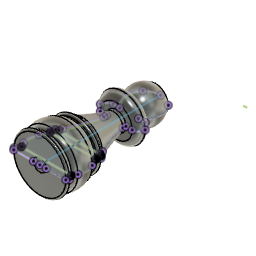
Pawn v1 (Autodesk Fusion 360 design; units mm, degrees)
Autodesk Fusion 360 part; units mm, degrees
sketch "SVG" plane through (0, 0, 0) normal (0, 0, 1) x (1, 0, 0)
  line L0 (6.638277, 6.628661) -> (13.5992, 6.628661)
  spline S0 degree 3 poles (13.5992, 6.628661) (13.764035, 6.697718) (13.883627, 6.821014) (13.840499, 7.032678) knots 0 0 0 0 1 1 1 1
  spline S1 degree 3 poles (13.840499, 7.032678) (13.797107, 7.245932) (13.689951, 7.340653) (13.552897, 7.384045) knots 0 0 0 0 1 1 1 1
  line L1 (13.552897, 7.384045) -> (6.732998, 7.384045)
  spline S2 degree 3 poles (6.732998, 7.384045) (6.567368, 7.312607) (6.482173, 7.158356) (6.47741, 6.931344) knots 0 0 0 0 1 1 1 1
  spline S3 degree 3 poles (6.47741, 6.931344) (6.473706, 6.755926) (6.539058, 6.6702) (6.638277, 6.628661) knots 0 0 0 0 1 1 1 1
  line L2 (6.393008, 2.442159) -> (13.837325, 2.442159)
  spline S4 degree 3 poles (13.837325, 2.442159) (14.039467, 2.558577) (14.139479, 2.79538) (14.237375, 3.040645) knots 0 0 0 0 1 1 1 1
  spline S5 degree 3 poles (14.237375, 3.040645) (14.557785, 3.840217) (14.452481, 4.624972) (14.138157, 5.390409) knots 0 0 0 0 1 1 1 1
  spline S6 degree 3 poles (14.138157, 5.390409) (13.977819, 5.780933) (13.813512, 6.179661) (13.492838, 6.478375) knots 0 0 0 0 1 1 1 1
  line L3 (13.492838, 6.478375) -> (6.728764, 6.478375)
  spline S7 degree 3 poles (6.728764, 6.478375) (6.705217, 6.464883) (6.683256, 6.447156) (6.663677, 6.421224) knots 0 0 0 0 1 1 1 1
  spline S8 degree 3 poles (6.663677, 6.421224) (5.92496, 5.438032) (5.450033, 4.392133) (5.901942, 3.132984) knots 0 0 0 0 1 1 1 1
  spline S9 degree 3 poles (5.901942, 3.132984) (6.059633, 2.693513) (6.152237, 2.513332) (6.393008, 2.442159) knots 0 0 0 0 1 1 1 1
  line L4 (13.857169, 2.29214) -> (6.251721, 2.29214)
  spline S10 degree 3 poles (6.251721, 2.29214) (5.976554, 2.202712) (5.81754, 1.928072) (5.850083, 1.583588) knots 0 0 0 0 1 1 1 1
  spline S11 degree 3 poles (5.850083, 1.583588) (5.886596, 1.196237) (6.201185, 1.374302) (6.371577, 1.372187) knots 0 0 0 0 1 1 1 1
  spline S12 degree 3 poles (6.371577, 1.372187) (7.901398, 1.354459) (9.431483, 1.363721) (10.961304, 1.365307) knots 0 0 0 0 1 1 1 1
  spline S13 degree 3 poles (10.961304, 1.365307) (11.987094, 1.365836) (13.013413, 1.37404) (14.039202, 1.365307) knots 0 0 0 0 1 1 1 1
  spline S14 degree 3 poles (14.039202, 1.365307) (14.29479, 1.362663) (14.34903, 1.449976) (14.296906, 1.687833) knots 0 0 0 0 1 1 1 1
  spline S15 degree 3 poles (14.296906, 1.687833) (14.222559, 2.028881) (14.119106, 2.199272) (13.857169, 2.29214) knots 0 0 0 0 1 1 1 1
  spline S16 degree 3 poles (11.453165, 12.878913) (11.390459, 13.146936) (11.38014, 13.267322) (11.475919, 13.320767) knots 0 0 0 0 1 1 1 1
  line L5 (11.475919, 13.320767) -> (12.455935, 13.320767)
  spline S17 degree 3 poles (12.455935, 13.320767) (13.013677, 13.320767) (13.46585, 13.77294) (13.46585, 14.330944) knots 0 0 0 0 1 1 1 1
  spline S18 degree 3 poles (13.46585, 14.330944) (13.46585, 14.888686) (13.013677, 15.341122) (12.455935, 15.341122) knots 0 0 0 0 1 1 1 1
  line L6 (12.455935, 15.341122) -> (11.438877, 15.341122)
  spline S19 degree 3 poles (11.438877, 15.341122) (11.429352, 15.344295) (11.420092, 15.346943) (11.410831, 15.350383) knots 0 0 0 0 1 1 1 1
  spline S20 degree 3 poles (11.410831, 15.350383) (13.075854, 16.539684) (12.898053, 18.449185) (11.933647, 19.477354) knots 0 0 0 0 1 1 1 1
  spline S21 degree 3 poles (11.933647, 19.477354) (11.002579, 20.469806) (9.249979, 20.579873) (8.185031, 19.460684) knots 0 0 0 0 1 1 1 1
  spline S22 degree 3 poles (8.185031, 19.460684) (7.351328, 18.58465) (6.960539, 16.736268) (8.722399, 15.341122) knots 0 0 0 0 1 1 1 1
  line L7 (8.722399, 15.341122) -> (7.647133, 15.341122)
  spline S23 degree 3 poles (7.647133, 15.341122) (7.089391, 15.341122) (6.636953, 14.888682) (6.636953, 14.330944) knots 0 0 0 0 1 1 1 1
  spline S24 degree 3 poles (6.636953, 14.330944) (6.636953, 13.77294) (7.089391, 13.320767) (7.647133, 13.320767) knots 0 0 0 0 1 1 1 1
  line L8 (7.647133, 13.320767) -> (8.59831, 13.320767)
  spline S25 degree 3 poles (8.59831, 13.320767) (8.788545, 13.257794) (8.759176, 13.091901) (8.647258, 12.651105) knots 0 0 0 0 1 1 1 1
  spline S26 degree 3 poles (8.647258, 12.651105) (8.233978, 11.020479) (7.806147, 9.394085) (7.164532, 7.83516) knots 0 0 0 0 1 1 1 1
  spline S27 degree 3 poles (7.164532, 7.83516) (7.101826, 7.683288) (7.115584, 7.616613) (7.183318, 7.58063) knots 0 0 0 0 1 1 1 1
  line L9 (7.183318, 7.58063) -> (13.14782, 7.58063)
  spline S28 degree 3 poles (13.14782, 7.58063) (13.248626, 7.655242) (13.202325, 7.751287) (13.083791, 8.027247) knots 0 0 0 0 1 1 1 1
  spline S29 degree 3 poles (13.083791, 8.027247) (12.407252, 9.599931) (11.845277, 11.211242) (11.453165, 12.878913) knots 0 0 0 0 1 1 1 1
  spline S30 degree 3 poles (18.34265, 25.31671) (18.224382, 25.33867) (18.094471, 25.302422) (17.970911, 25.289459) knots 0 0 0 0 1 1 1 1
  line L10 (9.96745, 20.259532) -> (9.96745, 1.363549)
  constraint perpendicular L4 L10
revolve "Revolve1" add sketch "SVG" angle 360 about axis through (9.96745, 20.259532, 0) along (0, -1, 0) contours L0 S0 S1 L1 L10 | L2 S4 S5 S6 L3 L10 | L4 S12 S13 S14 S15 L10 | S16 L5 S17 S18 L6 S19 S20 S21 L9 S28 S29 L10 picked at (12.373182, 6.880456) picked at (11.357685, 4.770315) picked at (11.595308, 1.983196) picked at (11.737686, 8.675112) makes body 1 at (11.280191, 6.628661, 0.862374) makes body 2 at (5.788284, 4.774023, -1.289102) makes body 3 at (12.419788, 9.613463, -0.369631) makes body 4 at (12.99814, 1.369306, -0.303266)
sketch "Pion" plane through (0, 0, 0) normal (0, 0, 1) x (1, 0, 0)
  spline S0 degree 3 poles (14.296906, 1.687833) (14.269631, 1.812951) (14.236651, 1.924427) (14.15614, 2.076533) (14.116832, 2.129723) (14.009728, 2.224115) (13.941741, 2.262156) (13.857169, 2.29214) knots -0.08939975 -0.08939975 -0.08939975 -0.08939975 -0.0516416 -0.0516416 -0.02691914 -0.02691914 0 0 0 0
  line L0 (13.857169, 2.29214) -> (6.077731, 2.29214)
  spline S1 degree 3 poles (6.077731, 2.29214) (6.018123, 2.271007) (5.960583, 2.243682) (5.861134, 2.172033) (5.821359, 2.131321) (5.719625, 1.986228) (5.675175, 1.858392) (5.637994, 1.687833) knots -0.10663916 -0.10663916 -0.10663916 -0.10663916 -0.07847511 -0.07847511 -0.05236952 -0.05236952 0 0 0 0
  spline S2 degree 3 poles (5.637994, 1.687833) (5.620994, 1.610259) (5.615328, 1.548816) (5.627557, 1.483197) (5.633268, 1.465739) (5.651293, 1.434659) (5.662703, 1.421924) (5.693629, 1.398463) (5.714663, 1.388482) (5.780478, 1.36961) (5.831783, 1.364646) (5.895698, 1.365307) knots -0.07987643 -0.07987643 -0.07987643 -0.07987643 -0.05202481 -0.05202481 -0.0414749 -0.0414749 -0.03139166 -0.03139166 -0.01917533 -0.01917533 0 0 0 0
  spline S3 degree 3 poles (5.895698, 1.365307) (6.408638, 1.369674) (6.921725, 1.369806) (7.947679, 1.367755) (8.460684, 1.365572) (8.973595, 1.365307) knots -0.30771325 -0.30771325 -0.30771325 -0.30771325 -0.15387332 -0.15387332 0 0 0 0
  spline S4 degree 3 poles (8.973595, 1.365307) (9.139235, 1.365136) (9.304876, 1.364874) (9.635567, 1.364259) (9.800634, 1.363907) (9.966264, 1.363551) (9.966857, 1.36355) (9.96745, 1.363549) knots -0.09919894 -0.09919894 -0.09919894 -0.09919894 -0.04951132 -0.04951132 0 0 0.00017787 0.00017787 0.00017787 0.00017787
  spline S5 degree 3 poles (9.96745, 1.363549) (9.968043, 1.36355) (9.968636, 1.363551) (10.134266, 1.363907) (10.299333, 1.364259) (10.630023, 1.364874) (10.795665, 1.365136) (10.961304, 1.365307) knots -0.09938539 -0.09938539 -0.09938539 -0.09938539 -0.09920751 -0.09920751 -0.04969191 -0.04969191 0 0 0 0
  spline S6 degree 3 poles (10.961304, 1.365307) (11.474215, 1.365572) (11.987221, 1.367755) (13.013175, 1.369806) (13.526262, 1.369674) (14.039202, 1.365307) knots -0.30780865 -0.30780865 -0.30780865 -0.30780865 -0.15388763 -0.15388763 0 0 0 0
  spline S7 degree 3 poles (14.039202, 1.365307) (14.074327, 1.364944) (14.112195, 1.366212) (14.176578, 1.37548) (14.203328, 1.382224) (14.242851, 1.40008) (14.258087, 1.409699) (14.283678, 1.4347) (14.293225, 1.449053) (14.308742, 1.485627) (14.313419, 1.50931) (14.316324, 1.578403) (14.309938, 1.628363) (14.296906, 1.687833) knots -0.08001679 -0.08001679 -0.08001679 -0.08001679 -0.06355834 -0.06355834 -0.04975587 -0.04975587 -0.03990536 -0.03990536 -0.03027504 -0.03027504 -0.01826445 -0.01826445 0 0 0 0
  spline S8 degree 3 poles (14.138157, 5.390409) (14.053933, 5.595547) (13.968609, 5.802964) (13.759865, 6.176143) (13.642707, 6.33877) (13.492838, 6.478375) knots -0.12796857 -0.12796857 -0.12796857 -0.12796857 -0.06144539 -0.06144539 0 0 0 0
  line L1 (13.492838, 6.478375) -> (6.442062, 6.478375)
  spline S9 degree 3 poles (6.442062, 6.478375) (6.284165, 6.331292) (6.162768, 6.15886) (5.95807, 5.782979) (5.876907, 5.58566) (5.796743, 5.390409) knots -0.12807049 -0.12807049 -0.12807049 -0.12807049 -0.06332025 -0.06332025 0 0 0 0
  spline S10 degree 3 poles (5.796743, 5.390409) (5.62307, 4.967483) (5.506569, 4.522493) (5.500445, 3.709827) (5.565678, 3.369664) (5.697524, 3.040645) knots -0.24362958 -0.24362958 -0.24362958 -0.24362958 -0.10633604 -0.10633604 0 0 0 0
  spline S11 degree 3 poles (5.697524, 3.040645) (5.766746, 2.86722) (5.837072, 2.697867) (5.988113, 2.520503) (6.038504, 2.476179) (6.097575, 2.442159) knots -0.06988605 -0.06988605 -0.06988605 -0.06988605 -0.02044994 -0.02044994 0 0 0 0
  line L2 (6.097575, 2.442159) -> (13.837325, 2.442159)
  spline S12 degree 3 poles (13.837325, 2.442159) (13.887664, 2.47115) (13.931836, 2.507702) (14.011586, 2.59368) (14.046091, 2.642386) (14.138963, 2.797517) (14.188442, 2.918051) (14.237375, 3.040645) knots -0.07769775 -0.07769775 -0.07769775 -0.07769775 -0.05882377 -0.05882377 -0.03959964 -0.03959964 0 0 0 0
  spline S13 degree 3 poles (14.237375, 3.040645) (14.314635, 3.233444) (14.369844, 3.432124) (14.43123, 3.833543) (14.438707, 4.030388) (14.399622, 4.629398) (14.290617, 5.019141) (14.138157, 5.390409) knots -0.24206707 -0.24206707 -0.24206707 -0.24206707 -0.17982962 -0.17982962 -0.12040588 -0.12040588 0 0 0 0
  line L3 (6.097575, 2.442159) -> (6.077731, 2.29214)
  line L4 (13.837325, 2.442159) -> (13.857169, 2.29214)
  spline S14 degree 3 poles (9.96745, 20.259532) (9.966566, 20.259564) (9.965682, 20.259595) (9.749904, 20.267162) (9.534261, 20.248772) (9.115206, 20.161638) (8.911934, 20.093397) (8.450603, 19.871433) (8.205829, 19.695418) (8.001252, 19.477354) knots -0.21837472 -0.21837472 -0.21837472 -0.21837472 -0.21810941 -0.21810941 -0.15361398 -0.15361398 -0.08970139 -0.08970139 0 0 0 0
  spline S15 degree 3 poles (8.001252, 19.477354) (7.832849, 19.297816) (7.690511, 19.093672) (7.462424, 18.650745) (7.377782, 18.410828) (7.261314, 17.841501) (7.254004, 17.509559) (7.366737, 16.849565) (7.488608, 16.533131) (7.888418, 15.889507) (8.18373, 15.593482) (8.524069, 15.350383) knots -0.47792048 -0.47792048 -0.47792048 -0.47792048 -0.40348961 -0.40348961 -0.32738532 -0.32738532 -0.22800437 -0.22800437 -0.12547317 -0.12547317 0 0 0 0
  spline S16 degree 3 poles (8.524069, 15.350383) (8.519455, 15.348669) (8.514853, 15.347156) (8.505499, 15.344169) (8.500762, 15.342701) (8.496023, 15.341122) knots -0.00301721 -0.00301721 -0.00301721 -0.00301721 -0.00149859 -0.00149859 0 0 0 0
  line L5 (8.496023, 15.341122) -> (7.478964, 15.341122)
  spline S17 degree 3 poles (7.478964, 15.341122) (7.408737, 15.341122) (7.338867, 15.333949) (7.203545, 15.305485) (7.138597, 15.284743) (6.954326, 15.204474) (6.84409, 15.127633) (6.662246, 14.938978) (6.590998, 14.829587) (6.49371, 14.589263) (6.46905, 14.461195) (6.46905, 14.330944) knots -0.15943999 -0.15943999 -0.15943999 -0.15943999 -0.13834264 -0.13834264 -0.1178842 -0.1178842 -0.07792732 -0.07792732 -0.03907516 -0.03907516 0 0 0 0
  spline S18 degree 3 poles (6.46905, 14.330944) (6.46905, 14.260636) (6.476228, 14.190684) (6.50472, 14.055211) (6.525478, 13.990206) (6.605763, 13.805909) (6.682562, 13.695703) (6.871116, 13.513919) (6.980432, 13.442703) (7.22067, 13.345423) (7.348724, 13.320767) (7.478964, 13.320767) knots -0.159448 -0.159448 -0.159448 -0.159448 -0.13832656 -0.13832656 -0.11784644 -0.11784644 -0.07790258 -0.07790258 -0.03907211 -0.03907211 0 0 0 0
  line L6 (7.478964, 13.320767) -> (8.458981, 13.320767)
  spline S19 degree 3 poles (8.458981, 13.320767) (8.471559, 13.313748) (8.482981, 13.305199) (8.502301, 13.284166) (8.509652, 13.272436) (8.52442, 13.237861) (8.529093, 13.211834) (8.531344, 13.110028) (8.513089, 13.012929) (8.481735, 12.878913) knots -0.08233592 -0.08233592 -0.08233592 -0.08233592 -0.0709606 -0.0709606 -0.05981326 -0.05981326 -0.04129035 -0.04129035 0 0 0 0
  spline S20 degree 3 poles (8.481735, 12.878913) (8.286062, 12.046705) (8.047743, 11.22706) (7.498562, 9.608277) (7.188763, 8.812159) (6.851109, 8.027247) knots -0.51280622 -0.51280622 -0.51280622 -0.51280622 -0.25633704 -0.25633704 0 0 0 0
  spline S21 degree 3 poles (6.851109, 8.027247) (6.816277, 7.946155) (6.788833, 7.883249) (6.750435, 7.782521) (6.738532, 7.744056) (6.731257, 7.692914) (6.730951, 7.675745) (6.73618, 7.645391) (6.741149, 7.632172) (6.75794, 7.605716) (6.77051, 7.592894) (6.78708, 7.58063) knots -0.03971602 -0.03971602 -0.03971602 -0.03971602 -0.02796391 -0.02796391 -0.01760702 -0.01760702 -0.01161353 -0.01161353 -0.00618442 -0.00618442 0 0 0 0
  line L7 (6.78708, 7.58063) -> (13.14782, 7.58063)
  spline S22 degree 3 poles (13.14782, 7.58063) (13.164779, 7.593182) (13.177549, 7.606319) (13.194296, 7.633335) (13.199117, 7.646711) (13.204562, 7.680752) (13.203278, 7.702757) (13.184269, 7.796254) (13.143074, 7.889229) (13.083791, 8.027247) knots -0.08957468 -0.08957468 -0.08957468 -0.08957468 -0.0748598 -0.0748598 -0.06212384 -0.06212384 -0.04506339 -0.04506339 0 0 0 0
  spline S23 degree 3 poles (13.083791, 8.027247) (12.746137, 8.812159) (12.436338, 9.608277) (11.887156, 11.22706) (11.648838, 12.046705) (11.453165, 12.878913) knots -0.51280921 -0.51280921 -0.51280921 -0.51280921 -0.25647068 -0.25647068 0 0 0 0
  spline S24 degree 3 poles (11.453165, 12.878913) (11.422467, 13.010123) (11.404325, 13.105947) (11.405315, 13.202996) (11.408426, 13.226155) (11.419573, 13.261277) (11.426582, 13.275419) (11.447378, 13.30167) (11.460732, 13.312293) (11.475919, 13.320767) knots -0.03234854 -0.03234854 -0.03234854 -0.03234854 -0.016268 -0.016268 -0.01002611 -0.01002611 -0.00521732 -0.00521732 0 0 0 0
  line L8 (11.475919, 13.320767) -> (12.455935, 13.320767)
  spline S25 degree 3 poles (12.455935, 13.320767) (12.526167, 13.320767) (12.596042, 13.327937) (12.731376, 13.356391) (12.796319, 13.377123) (12.980555, 13.457351) (13.090756, 13.534136) (13.272582, 13.7227) (13.343827, 13.832056) (13.441176, 14.072435) (13.46585, 14.200596) (13.46585, 14.330944) knots -0.15945093 -0.15945093 -0.15945093 -0.15945093 -0.13835207 -0.13835207 -0.11789128 -0.11789128 -0.07795013 -0.07795013 -0.03910464 -0.03910464 0 0 0 0
  spline S26 degree 3 poles (13.46585, 14.330944) (13.46585, 14.401253) (13.458665, 14.471205) (13.430153, 14.606683) (13.409377, 14.671706) (13.329038, 14.856035) (13.252188, 14.966266) (13.063578, 15.148041) (12.954261, 15.219246) (12.714087, 15.316478) (12.586105, 15.341122) (12.455935, 15.341122) knots -0.1594394 -0.1594394 -0.1594394 -0.1594394 -0.13831779 -0.13831779 -0.11783519 -0.11783519 -0.07787887 -0.07787887 -0.03905092 -0.03905092 0 0 0 0
  line L9 (12.455935, 15.341122) -> (11.438877, 15.341122)
  spline S27 degree 3 poles (11.438877, 15.341122) (11.434138, 15.342701) (11.429401, 15.344169) (11.420047, 15.347156) (11.415445, 15.348669) (11.410831, 15.350383) knots -0.00293383 -0.00293383 -0.00293383 -0.00293383 -0.00147665 -0.00147665 0 0 0 0
  spline S28 degree 3 poles (11.410831, 15.350383) (11.645945, 15.518321) (11.860748, 15.712359) (12.207852, 16.133121) (12.343652, 16.35031) (12.584139, 16.901557) (12.656816, 17.238822) (12.667886, 17.942441) (12.599849, 18.300924) (12.342675, 18.944962) (12.162117, 19.233778) (11.933647, 19.477354) knots -0.4732211 -0.4732211 -0.4732211 -0.4732211 -0.38716174 -0.38716174 -0.31060386 -0.31060386 -0.2076949 -0.2076949 -0.10018713 -0.10018713 0 0 0 0
  spline S29 degree 3 poles (11.933647, 19.477354) (11.729071, 19.695418) (11.484297, 19.871433) (11.022965, 20.093397) (10.819693, 20.161638) (10.400638, 20.248772) (10.184996, 20.267162) (9.969218, 20.259595) (9.968334, 20.259564) (9.96745, 20.259532) knots -0.2181513 -0.2181513 -0.2181513 -0.2181513 -0.12843268 -0.12843268 -0.06450781 -0.06450781 0 0 0.00026536 0.00026536 0.00026536 0.00026536
  spline S30 degree 3 poles (13.840499, 7.032678) (13.828926, 7.089556) (13.811089, 7.146494) (13.75964, 7.241592) (13.72929, 7.280083) (13.649736, 7.345195) (13.603201, 7.368119) (13.552897, 7.384045) knots -0.04831531 -0.04831531 -0.04831531 -0.04831531 -0.03083409 -0.03083409 -0.01582959 -0.01582959 0 0 0 0
  line L10 (13.552897, 7.384045) -> (6.382003, 7.384045)
  spline S31 degree 3 poles (6.382003, 7.384045) (6.339871, 7.370706) (6.300081, 7.352363) (6.226031, 7.299836) (6.194838, 7.266727) (6.136176, 7.176894) (6.11076, 7.113076) (6.0944, 7.032678) knots -0.06133384 -0.06133384 -0.06133384 -0.06133384 -0.04345228 -0.04345228 -0.02461374 -0.02461374 0 0 0 0
  spline S32 degree 3 poles (6.0944, 7.032678) (6.086593, 6.994362) (6.083333, 6.955086) (6.090361, 6.882387) (6.098813, 6.849932) (6.130592, 6.781579) (6.155628, 6.749038) (6.229053, 6.68119) (6.281718, 6.651276) (6.3357, 6.628661) knots -0.05190443 -0.05190443 -0.05190443 -0.05190443 -0.04017365 -0.04017365 -0.02999392 -0.02999392 -0.01755829 -0.01755829 0 0 0 0
  line L11 (6.3357, 6.628661) -> (13.5992, 6.628661)
  spline S33 degree 3 poles (13.5992, 6.628661) (13.642111, 6.646638) (13.684059, 6.669172) (13.752392, 6.721585) (13.780148, 6.749857) (13.822566, 6.815049) (13.836524, 6.849874) (13.852874, 6.935467) (13.850273, 6.984708) (13.840499, 7.032678) knots -0.05198256 -0.05198256 -0.05198256 -0.05198256 -0.03802361 -0.03802361 -0.02614297 -0.02614297 -0.01468671 -0.01468671 0 0 0 0
  line L12 (6.442062, 6.478375) -> (6.3357, 6.628661)
  line L13 (13.492838, 6.478375) -> (13.5992, 6.628661)
  line L14 (13.14782, 7.58063) -> (13.552897, 7.384045)
  line L15 (6.78708, 7.58063) -> (6.382003, 7.384045)
  line L16 (9.96745, 7.58063) -> (9.96745, 7.384045)
  line L17 (9.96745, 6.628661) -> (9.96745, 6.478375)
  line L18 (9.96745, 2.442159) -> (9.96745, 2.29214)
revolve "Revolve2" add sketch "Pion" angle 360 about axis through (9.96745, 2.442159, 0) along (0, -1, 0) contours L0 L2 L4 L18 picked at (12.553981, 2.342147) bodies 2 4
revolve "Revolve3" add sketch "Pion" angle 360 about axis through (9.96745, 6.628661, 0) along (0, -1, 0) contours L1 L11 L13 L17 | L7 L10 L14 L16 picked at (12.353162, 6.578566) picked at (12.222722, 7.449573) bodies 1 2 3
named bodies: "Pion"
